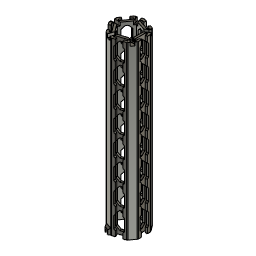
led-lamp-internal-frame (Autodesk Fusion 360 design; units mm, degrees)
Autodesk Fusion 360 part; units mm, degrees
note: some values were not read from the file. Set by a fixed rule: which sketch regions a step uses.
sketch "Sketch1" plane through (0, 0, 0) normal (0, 0, 1) x (1, 0, 0)
  line L0 (-13.6104, 0) -> (-4.2058, 12.9443)
  line L1 (-4.2058, 12.9443) -> (11.0111, 8)
  line L2 (11.0111, 8) -> (11.0111, -8)
  line L3 (-13.6104, 0) -> (-4.2058, -12.9443)
  line L4 (-4.2058, -12.9443) -> (11.0111, -8)
  line L5 (0, 0) -> (3.4026, 10.4721)
  line L6 (0, 0) -> (11.0111, 0)
  line L7 (15.5111, 6.5) -> (13.5111, 6.5)
  line L8 (13.5111, 6.5) -> (13.5111, -6.5)
  line L9 (13.5111, -6.5) -> (15.5111, -6.5)
  line L10 (15.5111, -6.5) -> (15.5111, -3.5)
  line L11 (15.5111, -3.5) -> (18.0111, -3.5)
  line L12 (18.0111, -3.5) -> (18.0111, -8)
  line L13 (18.0111, -8) -> (11.0111, -8)
  line L14 (18.0111, 8) -> (18.0111, 3.5)
  line L15 (18.0111, 3.5) -> (15.5111, 3.5)
  line L16 (15.5111, 3.5) -> (15.5111, 6.5)
  line L17 (17.5802, 8) -> (18.0111, 7.0305)
  line L18 (15.5111, 6.5) -> (17.7956, 7.5152)
  line L19 (17.5802, -8) -> (18.0111, -7.0305)
  line L20 (15.5111, -6.5) -> (17.7956, -7.5152)
  line L21 (17.5802, 8) -> (13.041, 14.2476)
  line L22 (13.041, 14.2476) -> (11.0111, 8)
  line L23 (11.0111, 8) -> (17.5802, 8)
  line L24 (17.5802, 8) -> (18.0111, 8)
  dimension "d5" = 108
  dimension "d6" = 108
  dimension "d8" = 16
  dimension "d10" = 13
  dimension "d11" = 3
  dimension "d12" = 2.5
  dimension "d13" = 2.5
  dimension "d16" = 2.5
  dimension "d17" = 2.5
  dimension "d18" = 2
  dimension "d33" = 72
  constraint equal L0 L1
  constraint equal L1 L2
  constraint equal L0 L3
  constraint equal L3 L4
  constraint coincident L5.start L6.start
  constraint midpoint L1 L5.end
  constraint midpoint L2 L6.end
  constraint equal L5 L6
  constraint perpendicular L2 L6
  constraint horizontal L6
  constraint perpendicular L8 L9
  constraint perpendicular L9 L10
  constraint perpendicular L10 L11
  constraint perpendicular L11 L12
  constraint perpendicular L12 L13
  constraint parallel L11 L15
  constraint collinear L10 L16
  constraint collinear L12 L14
  constraint coincident L2.end L4.end
  constraint equal L10 L16
  constraint equal L12 L14
  constraint coincident L14 L17.end
  constraint midpoint L17 L18.end
  constraint perpendicular L17 L18
  constraint midpoint L19 L20.end
  constraint coincident L13 L19.start
  constraint coincident L12 L19.end
  constraint perpendicular L19 L20
  constraint coincident L17.start L21.start
  constraint perpendicular L14 L24
  constraint perpendicular L7 L8
  constraint collinear L23 L24
  constraint equal L22 L23
  measures "d5" angle of L0 L3
  measures "d6" angle of L3 L4
  measures "d8" distance of L0.end L1.end
  measures "d10" distance of L7.end L8.end
  measures "d11" distance of L7.start L15.end
  measures "d12" distance of L14 L16
  measures "d13" distance of L2 L8
  measures "d16" distance of L7.start L18.end
  measures "d17" distance of L9.end L20.end
  measures "d18" distance of L8.end L9.end
  measures "d33" angle of L22 L23
extrude "Extrude1" add sketch "Sketch1" along normal blind 200 contours L2 L7 L8 L9 L13 L17 L18 L19 L20 L23 | L21 L22 L23 | L10 L11 L12 L19 L20 | L14 L15 L16 L17 L18 makes body 1
sketch "Sketch2" plane through (11.0111, 0, 0) normal (-1, 0, 0) x (0, -1, 0)
  line L0 (-8, 0) -> (8, 0)
  line L1 (8, 0) -> (8, 200)
  line L2 (8, 200) -> (-8, 200)
  line L3 (-5, 24.5) -> (5, 24.5)
  line L4 (5, 24.5) -> (5, 4)
  line L5 (5, 4) -> (-5, 4)
  line L6 (-5, 4) -> (-5, 24.5)
  line L7 (-5, 7.5) -> (-1.5, 4)
  line L8 (1.5, 4) -> (5, 7.5)
  line L9 (-5, 21) -> (-1.5, 24.5)
  line L10 (1.5, 24.5) -> (5, 21)
  line L11 (-5, 24.5) -> (-3.25, 22.75)
  line L12 (3.25, 22.75) -> (5, 24.5)
  line L13 (5, 4) -> (3.25, 5.75)
  line L14 (-5, 4) -> (-3.25, 5.75)
  line L15 (-8, 200) -> (-8, 0)
  dimension "d19" = 10
  dimension "d20" = 3
  dimension "d21" = 4
  dimension "d22" = 3
  dimension "d23" = 20.5
  dimension "d24" = 3
  constraint horizontal L3
  constraint vertical L4
  constraint horizontal L5
  constraint vertical L6
  constraint midpoint L9 L11.end
  constraint coincident L3 L9.end
  constraint coincident L6 L9.start
  constraint perpendicular L9 L11
  constraint coincident L3 L10.start
  constraint coincident L4 L10.end
  constraint midpoint L10 L12.start
  constraint perpendicular L10 L12
  constraint equal L9 L10
  constraint coincident L5 L7.end
  constraint coincident L6 L7.start
  constraint coincident L5 L8.start
  constraint coincident L4 L8.end
  constraint midpoint L8 L13.end
  constraint midpoint L7 L14.end
  constraint perpendicular L8 L13
  constraint perpendicular L7 L14
  constraint equal L7 L8
  measures "d19" distance of L3.start L3.end
  measures "d20" distance of L1 L4
  measures "d21" distance of L0 L5
  measures "d22" distance of L9.end L10.start
  measures "d23" distance of L3.end L4.end
  measures "d24" distance of L7.end L8.start
extrude "Extrude2" cut sketch "Sketch2" against normal through all contours L3 L4 L5 L6 L7 L8 L9 L10 bodies 1
pattern_linear "R-Pattern1" count 8 spacing 24.5 along (0, 0, 1) of "Extrude2"
sketch "Sketch10" plane through (0, 0, 200) normal (0, 0, 1) x (-1, 0, 0)
  line L0 (-11.0111, -8) -> (-11.0111, 8)
  line L1 (-11.0111, 8) -> (-17.5802, 8)
  line L2 (-17.5802, 8) -> (-18.0111, 7.0305)
  line L3 (-18.0111, 7.0305) -> (-18.0111, 3.5)
  line L4 (-18.0111, 3.5) -> (-15.5111, 3.5)
  line L5 (-15.5111, 3.5) -> (-15.5111, 6.5)
  line L6 (-15.5111, 6.5) -> (-13.5111, 6.5)
  line L7 (-13.5111, 6.5) -> (-13.5111, -6.5)
  line L8 (-13.5111, -6.5) -> (-15.5111, -6.5)
  line L9 (-15.5111, -6.5) -> (-15.5111, -3.5)
  line L10 (-15.5111, -3.5) -> (-18.0111, -3.5)
  line L11 (-18.0111, -3.5) -> (-18.0111, -7.0305)
  line L12 (-18.0111, -7.0305) -> (-17.5802, -8)
  line L13 (-11.0111, -5.5255) -> (-16.4821, -9.5114)
  line L14 (-11.0111, 5.5302) -> (-11.0111, 8)
  line L15 (-11.0111, 8) -> (-14.4198, 8)
  line L16 (-14.4198, 8) -> (-11.0111, 5.5302)
  line L17 (-12.0644, -11.2419) -> (-14.131, -12.7474)
  line L18 (-14.131, -12.7474) -> (-16.4821, -9.5114)
  line L19 (-17.5802, -8) -> (-13.041, -14.2476)
  line L20 (-11.0111, -5.5255) -> (-11.0111, -8)
  line L21 (-11.0111, -8) -> (-12.0644, -11.2419)
  line L22 (-13.041, -14.2476) -> (-11.0111, -8)
  line L23 (-11.0111, -8) -> (-12.1887, -6.3835)
  line L24 (-11.0111, -8) -> (-9.8334, -9.6165)
  line L25 (-9.8334, -9.6165) -> (-12.0644, -11.2419)
  line L26 (-11.0111, 8) -> (-12.1845, 6.3804)
  dimension "d58" = 72
  dimension "d60" = 2
  dimension "d61" = 2
  dimension "d62" = 2
  constraint coincident L0 L13.start
  constraint collinear L1 L15
  constraint collinear L0 L14
  constraint coincident L13.end L18.end
  constraint collinear L18 L19
  constraint parallel L13 L17
  constraint coincident L0.start L20.end
  constraint coincident L13.start L20.start
  constraint coincident L17.start L22
  constraint coincident L13 L23.end
  constraint perpendicular L13 L23
  constraint perpendicular L24 L25
  constraint collinear L23 L24
  constraint coincident L0.end L1.start
  constraint coincident L16 L26.end
  constraint perpendicular L16 L26
  measures "d58" angle of L13 L16
  measures "d60" distance of L0.start L23.end
  measures "d61" distance of L17 L0.start
  measures "d62" distance of L0.end L26.end
extrude "Extrude6" cut sketch "Sketch10" against normal blind 4 contours L0 L13 L20 L23 | L13 L17 L18 L19 L21 L22 L23 | L0 L14 L16 L26 | L1 L15 L16 L26 bodies 1
pattern_circular "C-Pattern1" count 5 over 360 about axis through (0, 0, 1.75) along (0, 0, 1) of bodies 1 makes body 2 at (2.9271, 10.6266, 1.3333) makes body 3 at (-9.202, 6.0676, 1.3333) makes body 4 at (-8.6142, -6.8766, 1.3333) makes body 5 at (3.8781, -10.3176, 1.3333)
sketch "Sketch4" plane through (0, 0, 0) normal (0, 0, -1) x (1, 0, 0)
  line L0 (-2.1759, 19.1919) -> (-9.5204, 16.8055)
  line L1 (-9.5204, 16.8055) -> (-10.4388, 16.2744)
  line L2 (-10.4388, 16.2744) -> (-12.514, 13.4182)
  line L3 (-12.514, 13.4182) -> (-10.4915, 11.9487)
  line L4 (-10.4915, 11.9487) -> (-8.7281, 14.3758)
  line L5 (-8.7281, 14.3758) -> (-7.1101, 13.2002)
  line L6 (-7.1101, 13.2002) -> (-14.7513, 2.683)
  line L7 (-14.7513, 2.683) -> (-16.3693, 3.8586)
  line L8 (-16.3693, 3.8586) -> (-14.606, 6.2856)
  line L9 (-14.606, 6.2856) -> (-16.6285, 7.7551)
  line L10 (-16.6285, 7.7551) -> (-18.7037, 4.8989)
  line L11 (-18.7037, 4.8989) -> (-18.925, 3.8613)
  line L12 (-18.925, 3.8613) -> (-13.6104, 0)
  line L13 (-13.6104, 0) -> (-4.2058, 12.9443)
  line L14 (-4.2058, 12.9443) -> (-2.1759, 19.1919)
  line L15 (-8.2258, 17.2262) -> (-3.4705, 18.7713)
  line L16 (-3.4705, 18.7713) -> (-4.0885, 20.6734)
  line L17 (-4.0885, 20.6734) -> (-8.8438, 19.1283)
  line L18 (-8.8438, 19.1283) -> (-8.2258, 17.2262)
  line L19 (-9.5204, 16.8055) -> (-8.2258, 17.2262)
  line L20 (-3.4705, 18.7713) -> (-2.1759, 19.1919)
  line L21 (-4.0885, 20.6734) -> (-2.129, 19.1968)
  line L22 (-8.8438, 19.1283) -> (-9.5612, 16.782)
  line L23 (-2.1759, 19.1919) -> (-1.1207, 19.3021)
  dimension "d34" = 5
  dimension "d37" = 2
  dimension "d42" = 35
  constraint parallel L15 L17
  constraint parallel L16 L18
  constraint perpendicular L15 L16
  constraint collinear L0 L15
  constraint coincident L0.end L1.start
  constraint coincident L0.start L14.end
  constraint equal L19 L20
  constraint coincident L1 L22.end
  constraint coincident L21.end L23
  constraint equal L21 L22
  measures "d34" distance of L16.end L17.end
  measures "d37" distance of L15.end L16.end
  measures "d42" angle of L16 L21
extrude "Extrude3" add sketch "Sketch4" against normal blind 7 contours L0 L16 L20 L21 L23 | L0 L15 L16 L17 L18 | L0 L1 L18 L19 L22 bodies 4 5
chamfer "Chamfer1" distance 2 angle 45 1 edges at (-6.4662, -19.9008, 7) on bodies 4
sketch "Sketch7" plane through (-6.4662, -19.9008, 0) normal (-0.309017, -0.951057, 0) x (0.951057, -0.309017, 0)
  line L0 (2.5, 5) -> (-2.5, 5)
  line L1 (-2.5, 5) -> (-2.5, 0)
  line L2 (-2.5, 0) -> (2.5, 0)
  line L3 (2.5, 0) -> (2.5, 5)
  line L4 (-1.75, 3) -> (1.75, 3)
  line L5 (1.75, 3) -> (1.75, 0)
  line L6 (1.75, 0) -> (-1.75, 0)
  line L7 (-1.75, 0) -> (-1.75, 3)
  line L8 (-2.5, 0) -> (-1.75, 0)
  line L9 (1.75, 0) -> (2.5, 0)
  dimension "d43" = 3.5
  dimension "d44" = 3
  constraint horizontal L4
  constraint vertical L5
  constraint horizontal L6
  constraint vertical L7
  constraint collinear L2 L6
  constraint coincident L1.end L2.start
  constraint coincident L2.end L3.start
  constraint equal L8 L9
  measures "d43" distance of L4.start L4.end
  measures "d44" distance of L4.end L5.end
extrude "Extrude4" cut sketch "Sketch7" against normal blind 3 contours L2 L4 L5 L6 L7 bodies 4
